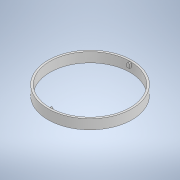
# Autodesk Inventor part: gripper_mount_ring
Saved by Autodesk Inventor 2022 (Build 260153000, 153)
## iProperties
Created: 2022-03-15
Part Number: gripper_mount_ring
Material: Generic
Document SubType Name: Modeling
Designer: kylem
Density: 1 g/cm^3
Appearance: Default
Author: kylem
Autodesk Inventor part; units mm, degrees
ref_plane "YZ Plane" through (0, 0, 0) normal (1, 0, 0) x (0, 1, 0)
ref_plane "XZ Plane" through (0, 0, 0) normal (0, 1, 0) x (-1, 0, 0)
ref_plane "XY Plane" through (0, 0, 0) normal (0, 0, 1) x (1, 0, 0)
sketch "Sketch1" plane through (0, 0, 0) normal (0, 1, 0) x (-1, 0, 0)
  circle A0 centre (0, 0) radius 65.5
  circle A1 centre (0, 0) radius 62.5
  dimension "d0" = 131
  dimension "d1" = 125
  constraints: 2 centre point, 2 coincident
  measures "d0" diameter of A0
  measures "d1" diameter of A1
extrude "Extrusion1" add sketch "Sketch1" along normal blind 15
sketch "Sketch2" plane through (0, 15, 0) normal (0, 1, 0) x (1, 0, 0)
  line L0 (0, 0) -> (1.9, 0)
  line L1 (1.9, 0) -> (-1.9, 0)
  line L2 (-1.9, 0) -> (-1.9, 75.6091)
  line L3 (-1.9, 75.6091) -> (1.9, 75.6091)
  line L4 (1.9, 75.6091) -> (1.9, 0)
  line L5 (1.9, 75.6091) -> (-1.9, 75.6091)
  line L6 (-1.9, 75.6091) -> (-1.9, -80.0242)
  line L7 (-1.9, -80.0242) -> (1.9, -80.0242)
  line L8 (1.9, -80.0242) -> (1.9, 75.6091)
  circle A0 centre (0, 0) radius 62.5 projected
  circle A1 centre (0, 0) radius 62.5
  circle A2 centre (0, 0) radius 59.5
  point P0 (-1.9, 59.4697)
  point P1 (1.9, 59.4697)
  point P2 (1.9, 62.4711)
  point P3 (-1.9, 62.4711)
  point P4 (1.9, -59.4697)
  point P5 (-1.9, -59.4697)
  point P6 (-1.9, -62.4711)
  point P7 (1.9, -62.4711)
  dimension "d4" = 1.9
  dimension "d5" = 3.8
  dimension "d6" = 3.8
  dimension "d7" = 119
  constraints: 18 end point, 4 parallel, 3 horizontal, 2 centre point, 2 coincident, 2 perpendicular
  measures "d4" distance of L0.start L0.end
  measures "d5" distance of L2.end L3.end
  measures "d6" distance of L7.end L6.end
  measures "d7" diameter of A2
extrude "Extrusion2" add sketch "Sketch2" against normal blind 7.5 contours A2 L2 A0 L4 | L8 A0 L6 A2
chamfer "Chamfer2" distance 1.8 angle 45 4 edges at (-1.9, 15, -60.9704) (1.9, 15, -60.9704) (-1.9, 15, 60.9704) (1.9, 15, 60.9704)
body "Solid1"
